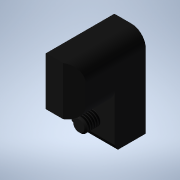
# Autodesk Inventor part: 686786 DGSL-12-AS
Saved by Autodesk Inventor 2021 (Build 250183000, 183)
## iProperties
Created: 2026-04-25
Part Number: 686786 DGSL-12-AS
Material: Generic
Catalog Web Link: www.3dfindit.com
Description: DGSL-(A)-stop
Vendor: FESTO
Document SubType Name: Modeling
Designer: psAdmin
Manufacturer: FESTO
Mass: 3.26091 g
Surface Area: 17.8066 cm^2
Volume: 3.26091 cm^3
Density: 1 g/cm^3
Appearance: PSOLRGB-128-128-128
Category: PARTsolutions
Company: FESTO
Title: 686786 DGSL-12
Author: Cadenas PARTsolutions
Comments: stop
PSOL_IDENT_0: {$CADENAS_DATA/23d-libs/festo/parts/d/dgsl/parts/dgsl_anschlag.prj},174 {VTYP=3D},{NB=686786 DGSL-12
PSOL_IDENT_1: -AS},{LINA=686786 DGSL-12},{NN=DGSL-(A)},{DATE=08.01.2026 09:12:23},{GEOMDATE=08.01.2026 09:12:00},{
PSOL_IDENT_2: VERSION=},{LINEID=130},{WBVAR=},{WBNUMERIC=}  {NB=686786 DGSL-12-AS},{LINA=686786 DGSL-12},{KT=DUMMY
PSOL_IDENT_3: },{TNR=686786},{TYP=DGSL-12},{KDM=16},{ANSCH=1.000},{B=12.000},{B4=6.000},{H=24.500},{H1=1.500},{H2=
PSOL_IDENT_4: 9.400},{H3=19.200},{H4=2.800},{H4B=11.000},{T=8.600},{T2=1.800},{T3=4.600},{T4=5.800},{D1=8.000},{D2=
PSOL_IDENT_5: 4.400},{R1=4.000},{R4=1.000},{W2=30.000},{AH1=11.000},{AH2=13.500},{AB1=8.800},{AB2=6.500},{AT1=19.0
PSOL_IDENT_6: 00},{AR1=2.400},{H16=5.200},{SW=3.000},{T5=0.000},{H5=0.000},{R5=0.000},{H6=0.000},{T6=2.300},{WK=60
PSOL_IDENT_7: .000},{R6=2.000},{SD=4.000},{SL=8.000},{SK=4.000},{SDK=7.000},{ST=2.000},{SV=0.400},{R100=0.600}
NB: 686786 DGSL-12-AS
NN: DGSL-(A)
NT: stop
NBSYN: $TNR. $TYP.-AS
LINA: 686786 DGSL-12
CATALOG: Festo
TNR: 686786
TYP: DGSL-12
KDM: 16
SW: 3
T5: 0
H5: 0
R5: 0
H6: 0
T6: 2.3
WK: 60
R6: 2
SD: 4
SL: 8
SK: 4
SDK: 7
ST: 2
SV: 0.4
R100: 0.6
SUPPLIER: FESTO
ARTICLENO: 686786 DGSL-12-AS
BOMINFO: 686786 DGSL-12
CREATOR: CADENAS GmbH
Autodesk Inventor part; units mm, degrees
sketch "Skizze_1" plane through (0, 0, 0) normal (0, 0, 1) x (1, 0, 0)
  line L0 (-6, 20.5) -> (-6, 0)
  line L1 (-6, 0) -> (6, 0)
  line L2 (6, 0) -> (6, 20.5)
  arc A0 (6, 20.5) -> (2, 24.5) centre (2, 20.5) ccw
  line L3 (2, 24.5) -> (-2, 24.5)
  arc A1 (-2, 24.5) -> (-6, 20.5) centre (-2, 20.5) ccw
  constraints: 8 end point, 4 point on circle, 2 centre point
extrude "Extrusion1" add sketch "Skizze_1" along normal blind 19
sketch "Skizze_2" plane through (0, 0, 0) normal (1, 0, 0) x (0, 1, 0)
  line L0 (1.5, 8.6) -> (0, 8.6)
  line L1 (0, 8.6) -> (0, 7.734)
  line L2 (0, 7.734) -> (1.5, 8.6)
  constraints: 6 end point
extrude "Extrusion2" cut sketch "Skizze_2" along normal mid plane 12
sketch "Skizze_5" plane through (0, 0, 0) normal (1, 0, 0) x (0, 1, 0)
  line L0 (5.2, 0) -> (5.2, 8.6)
  line L1 (5.2, 0.6) -> (8.3, 0.6)
  line L2 (8.3, 0.6) -> (8.7, 1)
  line L3 (8.7, 1) -> (8.7, 4.6)
  line L4 (8.7, 4.6) -> (9.2, 4.6)
  line L5 (9.2, 4.6) -> (9.2, 0)
  line L6 (9.2, 0) -> (5.2, 0)
  line L7 (5.2, 0) -> (5.2, 0.6)
  constraints: 16 end point
sketch "Sketch_1" plane through (0, 0, 8.6) normal (0, 0, 1) x (1, 0, 0)
  line L0 (-6, 24.5) -> (-6, 0)
  line L1 (-6, 0) -> (8, 0)
  line L2 (8, 0) -> (8, 15)
  line L3 (8, 15) -> (6, 15)
  arc A0 (2, 11) -> (6, 15) centre (2, 15) ccw
  line L4 (2, 11) -> (-2.8, 11)
  line L5 (-2.8, 11) -> (-2.8, 24.5)
  line L6 (-2.8, 24.5) -> (-6, 24.5)
  constraints: 14 end point, 2 point on circle, 1 centre point
extrude "Extrusion3" cut sketch "Sketch_1" along normal blind 19.8
revolve "Revolution1" cut sketch "Skizze_5" angle 360 about axis through (0, 5.2, 0) along (0, 0, -1)
sketch "Skizze_6" plane through (0, 5.2, 0.6) normal (0, 0, -1) x (0, 1, 0)
  line L0 (-1.5, -0.866) -> (0, -1.7321)
  line L1 (0, -1.7321) -> (1.5, -0.866)
  line L2 (1.5, -0.866) -> (1.5, 0.866)
  line L3 (1.5, 0.866) -> (0, 1.7321)
  line L4 (0, 1.7321) -> (-1.5, 0.866)
  line L5 (-1.5, 0.866) -> (-1.5, -0.866)
  constraints: 12 end point
extrude "Extrusion4" cut sketch "Skizze_6" against normal blind 2
sketch "Skizze_9" plane through (0, 0, 6.45) normal (0, 0, 1) x (1, 0, 0)
  line L0 (-6, 13.5) -> (-5.2, 13.5)
  arc A0 (-5.2, 13.5) -> (-2.8, 15.9) centre (-5.2, 15.9) ccw
  line L1 (-2.8, 15.9) -> (-2.8, 24.5)
  line L2 (-2.8, 24.5) -> (-6, 24.5)
  line L3 (-6, 24.5) -> (-6, 13.5)
  constraints: 8 end point, 2 point on circle, 1 centre point
extrude "Extrusion5" cut sketch "Skizze_9" along normal mid plane 12.9
sketch "Skizze_13" plane through (0, 0, 0) normal (1, 0, 0) x (0, 1, 0)
  line L0 (10.9, 10.9196) -> (10.9, 8.6)
  line L1 (10.9, 8.6) -> (11.2, 8.6)
  arc A0 (11.2, 8.6) -> (11.7196, 9.5) centre (11.2, 9.2) ccw
  line L2 (11.7196, 9.5) -> (10.9, 10.9196)
  constraints: 6 end point, 2 point on circle, 1 centre point
extrude "Extrusion6" cut sketch "Skizze_13" along normal mid plane 12
sketch "Sketch_3" plane through (0, 0, 0) normal (0, 1, 0) x (-1, 0, 0)
  line L0 (-2.0163, 19) -> (-6, 19)
  line L1 (-6, 19) -> (-6, 16.7)
  line L2 (-6, 16.7) -> (-2.0163, 19)
  constraints: 6 end point
extrude "Extrusion7" cut sketch "Sketch_3" along normal mid plane 49
sketch "Sketch_5" plane through (0, 0, 0) normal (1, 0, 0) x (0, 1, 0)
  line L0 (5.2, 8.6) -> (5.2, 12.6)
  line L1 (5.2, 12.6) -> (6.7705, 12.6)
  line L2 (6.7705, 12.6) -> (7.2, 12.1705)
  line L3 (7.2, 12.1705) -> (7.2, 8.6)
  line L4 (7.2, 8.6) -> (5.2, 8.6)
  line L5 (5.2, 8.6) -> (5.2, 12.6)
  constraints: 12 end point
revolve "Revolution2" add sketch "Sketch_5" angle 360 about axis through (0, 5.2, 8.6) along (0, 0, -1)
thread "Thread1" size "M4x0.7" class "6g" standard "ISO Metric profile" full length
ref_plane "ANBAU_XY" through (0, 5.2, 8.6) normal (0, 0, -1) x (1, 0, 0)
ref_plane "ANBAU_YZ" through (0, 5.2, 8.6) normal (1, 0, 0) x (0, -1, 0)
ref_plane "ANBAU_ZX" through (0, 5.2, 8.6) normal (0, -1, 0) x (0, 0, -1)
body "Solid1"
